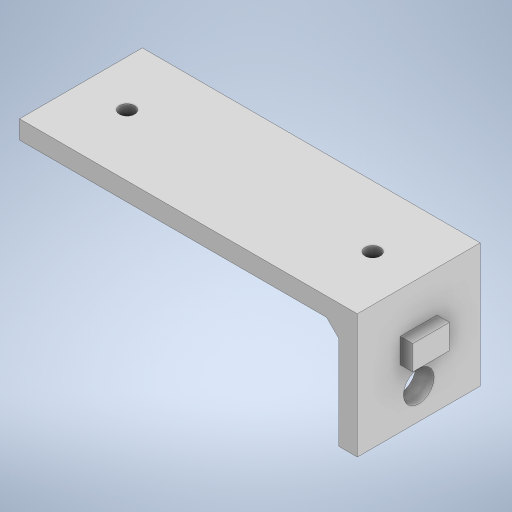
# Autodesk Inventor part: base
Saved by Autodesk Inventor 2024 (Build 280153000, 153)
## iProperties
Created: 2024-07-02
Part Number: base
Material: 일반
Document SubType Name: Modeling
Designer: Gihyeok Na
Density: 1 g/cm^3
Appearance: 기본값
Author: Gihyeok Na
Autodesk Inventor part; units mm, degrees
ref_plane "YZ Plane" through (0, 0, 0) normal (1, 0, 0) x (0, 1, 0)
ref_plane "XZ Plane" through (0, 0, 0) normal (0, 1, 0) x (-1, 0, 0)
ref_plane "XY Plane" through (0, 0, 0) normal (0, 0, 1) x (1, 0, 0)
sketch "스케치1" plane through (0, 0, 0) normal (0, 1, 0) x (-1, 0, 0)
  line L0 (-27.5, 10) -> (27.5, 10)
  line L1 (27.5, 10) -> (27.5, -10)
  line L2 (27.5, -10) -> (-27.5, -10)
  line L3 (-27.5, -10) -> (-27.5, 10)
  line L4 (-27.5, 10) -> (27.5, -10) construction
  line L5 (27.5, 10) -> (-27.5, -10) construction
  line L6 (-27.5, 10) -> (-24.5, 10)
  line L7 (-24.5, 10) -> (-24.5, -10)
  line L8 (-24.5, -10) -> (-27.5, -10)
  line L9 (-27.5, -10) -> (-27.5, 10)
  circle A0 centre (20, 0) radius 1.25
  circle A1 centre (-20, 0) radius 1.25
  point P0 (0, 0)
  dimension "d0" = 55
  dimension "d1" = 20
  dimension "d5" = 3
  dimension "d14" = 2.5
  dimension "d15" = 2.5
  dimension "d17" = 47.5
  dimension "d18" = 7.5
  constraints: 20 end point, 4 parallel, 2 centre point, 2 horizontal, 2 midpoint, 2 perpendicular, 1 point on line
  measures "d0" distance of L0.start L0.end
  measures "d1" distance of L0.end L1.end
  measures "d5" distance of L7.end L8.end
  measures "d14" diameter of A0
  measures "d15" diameter of A1
  measures "d17" distance from line of L3 A0.centre
  measures "d18" distance from line of L3 A1.centre
extrude "돌출1" add sketch "스케치1" along normal blind 3
extrude "돌출2" add sketch "스케치1" against normal blind 17.2 contours L0 L7 L2 L3
sketch "스케치2" plane through (24.5, -17.2, -10) normal (-1, 0, 0) x (0, 0, 1)
  line L0 (20, 17.2) -> (20, 0) projected
  line L1 (0, 17.2) -> (20, 17.2) projected
  line L2 (0, 17.2) -> (0, 0) projected
  line L3 (20, 0) -> (0, 0) projected
  line L4 (20, 17.2) -> (20, 0) projected
  circle A0 centre (10, 5) radius 2.5
  circle A1 centre (10, 5) radius 3.5
  point P0 (10, 17.2)
  point P1 (10, 0)
  dimension "d8" = 5
  dimension "d9" = 5
  dimension "d10" = 7
  constraints: 2 centre point, 1 coincident, 1 midpoint
  measures "d8" diameter of A0
  measures "d9" distance of point (10, 0) A0.centre
  measures "d10" diameter of A1
chamfer "모따기1" distance 2 angle 45 1 edges at (24.5, 0, 0)
extrude "돌출3" cut sketch "스케치2" against normal blind 3 contours A0
sketch "스케치5" plane through (27.5, 3, 10) normal (1, 0, 0) x (0, 0, -1)
  line L0 (0, -20.2) -> (0, 0) projected
  line L1 (20, -20.2) -> (0, -20.2) projected
  line L2 (7, -10.7) -> (13, -10.7)
  line L3 (20, -20.2) -> (20, 0) projected
  line L4 (10, -3) -> (10, -10.7) construction
  line L5 (7, -10.7) -> (7, -6.7)
  line L6 (13, -10.7) -> (13, -6.7)
  line L7 (7, -6.7) -> (13, -6.7)
  line L8 (20, -6.7) -> (20.03, -6.7)
  point P0 (7, -8.7)
  dimension "d33" = 3
  constraints: 12 end point, 3 horizontal, 2 midpoint, 2 perpendicular, 2 symmetric about line, 1 point on line
  measures "d33" distance from line of L4 point (7, -8.7)
extrude "돌출5" add sketch "스케치5" along normal blind 2
